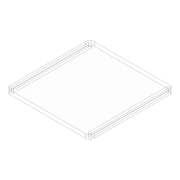
# Autodesk Inventor part: Adult fly trap top and bottom
Saved by Autodesk Inventor 2020 (Build 240168000, 168)
## iProperties
Created: 2020-09-12
Part Number: Adult fly trap top and bottom
Material: Generic
Document SubType Name: Modeling
Designer: ferrerx
Density: 1 g/cm^3
Appearance: Clear - Light
Author: ferrerx
Autodesk Inventor part; units mm, degrees
ref_plane "YZ Plane" through (0, 0, 0) normal (1, 0, 0) x (0, 1, 0)
ref_plane "XZ Plane" through (0, 0, 0) normal (0, 1, 0) x (-1, 0, 0)
ref_plane "XY Plane" through (0, 0, 0) normal (0, 0, 1) x (1, 0, 0)
sketch "Sketch1" plane through (0, 0, 0) normal (0, 1, 0) x (-1, 0, 0)
  line L0 (0, 0) -> (105, 0)
  line L1 (105, 0) -> (105, -105)
  line L2 (105, -105) -> (0, -105)
  line L3 (0, -105) -> (0, 0)
  dimension "d0" = 105
  dimension "d1" = 105
  constraints: 8 end point, 2 parallel, 1 horizontal, 1 perpendicular
  measures "d0" distance of L1.end L2.end
  measures "d1" distance of L2.end L0.start
extrude "Extrusion1" add sketch "Sketch1" along normal blind 5
fillet "Fillet1" radius 5 4 edges at (-105, 2.5, -105) (0, 2.5, 0) (0, 2.5, -105) (-105, 2.5, 0)
sketch "Sketch3" plane through (0, 5, 0) normal (0, 1, 0) x (1, 0, 0)
  line L0 (-102.5, 102.5) -> (-2.5, 102.5) construction
  line L1 (-2.5, 102.5) -> (-2.5, 2.5) construction
  line L2 (-2.5, 2.5) -> (-102.5, 2.5) construction
  line L3 (-102.5, 2.5) -> (-102.5, 102.5) construction
  line L4 (0, 5) -> (0, 100) projected
  line L5 (-5, 105) -> (-100, 105) projected
  line L6 (-105, 100) -> (-105, 5) projected
  line L7 (-100, 0) -> (-5, 0) projected
  point P0 (0, 0)
  dimension "d11" = 2.5
  dimension "d12" = 2.5
  dimension "d13" = 2.5
  dimension "d14" = 2.5
  constraints: 8 end point, 2 parallel, 1 horizontal, 1 perpendicular
  measures "d11" distance between parallel lines of L4 L1
  measures "d12" distance between parallel lines of L5 L0
  measures "d13" distance between parallel lines of L6 L3
  measures "d14" distance between parallel lines of L7 L2
sketch "Sketch4" plane through (0, 5, 0) normal (0, 1, 0) x (1, 0, 0)
  line L0 (-101, 101) -> (-4, 101) construction
  line L1 (-4, 101) -> (-4, 4) construction
  line L2 (-4, 4) -> (-101, 4) construction
  line L3 (-101, 4) -> (-101, 101) construction
  line L4 (0, 5) -> (0, 100) projected
  line L5 (-105, 100) -> (-105, 5) projected
  line L6 (-100, 0) -> (-5, 0) projected
  line L7 (-5, 105) -> (-100, 105) projected
  circle A0 centre (-101, 101) radius 1.5
  circle A1 centre (-4, 101) radius 1.5
  circle A2 centre (-4, 4) radius 1.5
  circle A3 centre (-101, 4) radius 1.5
  point P0 (0, 0)
  dimension "d15" = 4
  dimension "d16" = 4
  dimension "d17" = 4
  dimension "d18" = 4
  dimension "d19" = 3
  dimension "d20" = 3
  dimension "d21" = 3
  dimension "d22" = 3
  constraints: 8 end point, 4 centre point, 4 coincident, 2 parallel, 1 horizontal, 1 perpendicular
  measures "d15" distance between parallel lines of L4 L1
  measures "d16" distance between parallel lines of L5 L3
  measures "d17" distance between parallel lines of L6 L2
  measures "d18" distance between parallel lines of L7 L0
  measures "d19" diameter of A0
  measures "d20" diameter of A1
  measures "d21" diameter of A2
  measures "d22" diameter of A3
extrude "Extrusion3" cut sketch "Sketch4" against normal blind 10
sketch "Sketch5" plane through (0, 5, 0) normal (0, 1, 0) x (1, 0, 0)
  circle A0 centre (-4, 4) radius 1.5 projected
  line L0 (-5.5, 4) -> (-5.5, 101)
  circle A1 centre (-4, 101) radius 1.5 projected
  line L1 (-2.5, 101) -> (-2.5, 4)
  circle A2 centre (-101, 4) radius 1.5 projected
  circle A3 centre (-101, 101) radius 1.5 projected
  point P0 (0, 0)
  constraints: 4 end point, 4 point on circle, 1 tangent, 1 vertical
extrude "Extrusion4" cut sketch "Sketch5" against normal blind 10 contours A0 | A0 L0 A1 L1 | A1
ref_plane "Work Plane1" through (-52.5, 0, -5) normal (1, 0, 0) x (0, 0, -1)
mirror "Mirror1" about plane through (-52.5, 0, -5) normal (1, 0, 0) of "Extrusion4"
body "Solid1"
